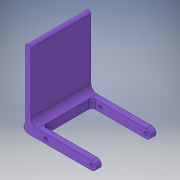
# Autodesk Inventor part: Mouth-Height-Lever-front
Saved by Autodesk Inventor 2018.3 (Build 223284000, 284)
## iProperties
Created: 2018-05-17
Part Number: Mouth-Height-Lever-front
Material: Generisch
Document SubType Name: Modeling
Designer: JochenAlt
Density: 1 g/cm^3
Appearance: Violett
Author: JochenAlt
Autodesk Inventor part; units mm, degrees
ref_plane "YZ Plane" through (0, 0, 0) normal (1, 0, 0) x (0, 1, 0)
ref_plane "XZ Plane" through (0, 0, 0) normal (0, 1, 0) x (-1, 0, 0)
ref_plane "XY Plane" through (0, 0, 0) normal (0, 0, 1) x (1, 0, 0)
sketch "Skizze4" plane through (0, 0, 0) normal (0, 1, 0) x (-1, 0, 0)
  line L0 (-38.5, 2.5) -> (-2.5, 2.5) construction
  line L1 (0, -11.3) -> (0, 50.3) construction
  line L2 (-49.2, 0) -> (8.2, 0) construction
  circle A0 centre (-38.5, 0) radius 2.5
  circle A1 centre (-38.5, 0) radius 1
  circle A2 centre (-2.5, 0) radius 2.5
  line L3 (-2.5, -2.5) -> (-38.5, -2.5) construction
  circle A3 centre (-12.5, 0) radius 2.5
  line L4 (-38.5, 2.5) -> (-12.5, 2.5)
  line L5 (-38.5, -2.5) -> (-12.5, -2.5)
  line L6 (-1, 2) -> (-1, 40)
  arc A4 (-1, 40) -> (-4, 40) centre (-2.5, 40) ccw
  circle A5 centre (-12.5, 0) radius 1
  line L7 (-4, 6.1116) -> (-4, 40)
  line L8 (-7.6116, 2.5) -> (-2.5, 2.5)
  line L9 (-7.6116, 2.5) -> (-7.6116, -2.5)
  line L10 (-7.6116, -2.5) -> (-2.5, -2.5)
  line L11 (-2.5, 0) -> (-2.5, 40) construction
  line L12 (-4, 6.1116) -> (-4, 2.5)
  line L13 (-7.6116, 2.5) -> (-12.5, 2.5)
  line L14 (-7.6116, -2.5) -> (-12.5, -2.5)
  arc A6 (-7.6116, 2.5) -> (-4, 6.1116) centre (-7.6116, 6.1116) ccw
  line L15 (-4, 2.5) -> (-4, 2)
  point P0 (0, 0)
  point P1 (-12.5, -2.5)
  dimension "d28" = 2
  dimension "d30" = 10
  dimension "d32" = 26
  dimension "d33" = 5
  dimension "d35" = 5
  dimension "d41" = 3
  dimension "d43" = 40
  constraints: 28 end point, 20 point on circle, 13 tangent, 7 centre point, 4 parallel, 4 vertical, 3 horizontal, 2 coincident, 1 equal radius, 1 point on line, 1 other
  measures "d28" diameter of A1
  measures "d30" distance of L11.start A3.centre
  measures "d32" distance of A3.centre A0.centre
  measures "d33" distance between parallel lines of L5 L4
  measures "d35" diameter of A2
  measures "d41" distance between parallel lines of L6 L7
  measures "d43" distance from line of L2 L11.end
extrude "Extrusion6" add sketch "Skizze4" along normal mid plane 34
extrude "Extrusion7" cut sketch "Skizze4" along normal mid plane 28 contours A0 | A0 L4 A3 L5 | L13 L9 L14 A3 | A3 | A1
fillet "Rundung3" radius 2 2 edges at (7.6116, 14, 0) (7.6116, -14, 0)
